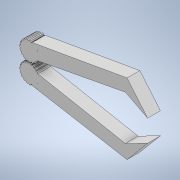
# Autodesk Inventor part: Claw(2 gear)
Saved by Autodesk Inventor 2021 (Build 250183000, 183)
## iProperties
Created: 2022-03-06
Part Number: Claw(2 gear)
Material: Generic
Document SubType Name: Modeling
Designer: Pradeep
Density: 1 g/cm^3
Appearance: Default
Author: Pradeep
Autodesk Inventor part; units mm, degrees
ref_plane "YZ Plane" through (0, 0, 0) normal (1, 0, 0) x (0, 1, 0)
ref_plane "XZ Plane" through (0, 0, 0) normal (0, 1, 0) x (-1, 0, 0)
ref_plane "XY Plane" through (0, 0, 0) normal (0, 0, 1) x (1, 0, 0)
sketch "Sketch1" plane through (0, 0, 0) normal (0, 0, 1) x (1, 0, 0)
  line L0 (36.6027, 32.7929) -> (34.9871, 31.7929)
  line L1 (34.9871, 29.7929) -> (34.9871, 31.7929)
  line L2 (34.9871, 29.7929) -> (36.6027, 28.7929)
  line L3 (36.6767, 28.3494) -> (35.4733, 26.879)
  line L4 (36.1227, 24.9874) -> (35.4733, 26.879)
  line L5 (36.1227, 24.9874) -> (37.9755, 24.5661)
  line L6 (38.1895, 24.1708) -> (37.5287, 22.3893)
  line L7 (38.7572, 20.811) -> (37.5287, 22.3893)
  line L8 (38.7572, 20.811) -> (40.6463, 21.0142)
  line L9 (40.9771, 20.7097) -> (40.9306, 18.8102)
  line L10 (42.6049, 17.7163) -> (40.9306, 18.8102)
  line L11 (42.6049, 17.7163) -> (44.3257, 18.5219)
  line L12 (44.7374, 18.3413) -> (45.3102, 16.5297)
  line L13 (47.249, 16.0387) -> (45.3102, 16.5297)
  line L14 (47.249, 16.0387) -> (48.615, 17.3594)
  line L15 (49.0631, 17.3223) -> (50.1931, 15.7948)
  line L16 (52.1862, 15.9599) -> (50.1931, 15.7948)
  line L17 (52.1862, 15.9599) -> (53.0494, 17.6526)
  line L18 (53.4852, 17.7629) -> (55.05, 16.6851)
  line L19 (56.8815, 17.4885) -> (55.05, 16.6851)
  line L20 (56.8815, 17.4885) -> (57.1483, 19.3697)
  line L21 (57.5247, 19.6156) -> (59.3546, 19.1043)
  line L22 (60.8261, 20.4588) -> (59.3546, 19.1043)
  line L23 (60.8261, 20.4588) -> (60.4676, 22.3247)
  line L24 (60.7437, 22.6795) -> (62.6405, 22.79)
  line L25 (63.5924, 24.549) -> (62.6405, 22.79)
  line L26 (63.5924, 24.549) -> (62.6475, 26.1974)
  line L27 (62.7935, 26.6226) -> (64.5516, 27.3431)
  line L28 (64.8808, 29.3158) -> (64.5516, 27.3431)
  line L29 (64.8808, 29.3158) -> (63.4519, 30.5681)
  line L30 (63.4519, 31.0176) -> (64.8808, 32.2699)
  line L31 (64.5516, 34.2426) -> (64.8808, 32.2699)
  line L32 (64.5516, 34.2426) -> (62.7935, 34.9631)
  line L33 (62.6475, 35.3883) -> (63.5924, 37.0367)
  line L34 (62.6405, 38.7957) -> (63.5924, 37.0367)
  line L35 (62.6405, 38.7957) -> (60.7437, 38.9062)
  line L36 (60.4676, 39.261) -> (60.8261, 41.1269)
  line L37 (59.3546, 42.4814) -> (60.8261, 41.1269)
  line L38 (59.3546, 42.4814) -> (57.5247, 41.9701)
  line L39 (57.1483, 42.216) -> (56.8815, 44.0972)
  line L40 (55.05, 44.9006) -> (56.8815, 44.0972)
  line L41 (55.05, 44.9006) -> (53.4852, 43.8228)
  line L42 (53.0494, 43.9331) -> (52.1862, 45.6258)
  line L43 (50.1931, 45.7909) -> (52.1862, 45.6258)
  line L44 (50.1931, 45.7909) -> (49.0631, 44.2634)
  line L45 (48.615, 44.2263) -> (47.249, 45.547)
  line L46 (45.3102, 45.056) -> (47.249, 45.547)
  line L47 (45.3102, 45.056) -> (44.7374, 43.2444)
  line L48 (44.3257, 43.0638) -> (42.6049, 43.8694)
  line L49 (40.9306, 42.7755) -> (42.6049, 43.8694)
  line L50 (40.9306, 42.7755) -> (40.9771, 40.876)
  line L51 (40.6463, 40.5715) -> (38.7572, 40.7747)
  line L52 (37.5287, 39.1964) -> (38.7572, 40.7747)
  line L53 (37.5287, 39.1964) -> (38.1895, 37.4149)
  line L54 (37.9755, 37.0196) -> (36.1227, 36.5983)
  line L55 (35.4733, 34.7067) -> (36.1227, 36.5983)
  line L56 (35.4733, 34.7067) -> (36.6767, 33.2363)
  arc A0 (40.9771, 40.876) -> (40.6463, 40.5715) centre (49.9537, 30.7929) ccw
  arc A1 (44.7374, 43.2444) -> (44.3257, 43.0638) centre (49.9537, 30.7929) ccw
  arc A2 (49.0631, 44.2634) -> (48.615, 44.2263) centre (49.9537, 30.7929) ccw
  arc A3 (53.4852, 43.8228) -> (53.0494, 43.9331) centre (49.9537, 30.7929) ccw
  arc A4 (57.5247, 41.9701) -> (57.1483, 42.216) centre (49.9537, 30.7929) ccw
  arc A5 (60.7437, 38.9062) -> (60.4676, 39.261) centre (49.9537, 30.7929) ccw
  arc A6 (62.7935, 34.9631) -> (62.6475, 35.3883) centre (49.9537, 30.7929) ccw
  arc A7 (63.4519, 30.5681) -> (63.4519, 31.0176) centre (49.9537, 30.7929) ccw
  arc A8 (62.6475, 26.1974) -> (62.7935, 26.6226) centre (49.9537, 30.7929) ccw
  arc A9 (60.4676, 22.3247) -> (60.7437, 22.6795) centre (49.9537, 30.7929) ccw
  arc A10 (57.1483, 19.3697) -> (57.5247, 19.6156) centre (49.9537, 30.7929) ccw
  arc A11 (53.0494, 17.6526) -> (53.4852, 17.7629) centre (49.9537, 30.7929) ccw
  arc A12 (48.615, 17.3594) -> (49.0631, 17.3223) centre (49.9537, 30.7929) ccw
  arc A13 (44.3257, 18.5219) -> (44.7374, 18.3413) centre (49.9537, 30.7929) ccw
  arc A14 (40.6463, 21.0142) -> (40.9771, 20.7097) centre (49.9537, 30.7929) ccw
  arc A15 (37.9755, 24.5661) -> (38.1895, 24.1708) centre (49.9537, 30.7929) ccw
  arc A16 (36.6027, 28.7929) -> (36.6767, 28.3494) centre (49.9537, 30.7929) ccw
  arc A17 (38.1895, 37.4149) -> (37.9755, 37.0196) centre (49.9537, 30.7929) ccw
  arc A18 (36.6767, 33.2363) -> (36.6027, 32.7929) centre (49.9537, 30.7929) ccw
  arc A19 (37.5287, 22.3893) -> (38.2823, 21.3706) centre (49.9537, 30.7929) ccw
  arc A20 (63.5924, 37.0367) -> (62.6405, 38.7957) centre (49.9537, 30.7929) ccw
  arc A21 (41.5275, 43.2025) -> (40.9306, 42.7755) centre (49.9537, 30.7929) ccw
  line L57 (55.05, 44.9006) -> (202.7711, 70.9478)
  line L58 (202.7711, 70.9478) -> (234.9105, 32.6456)
  line L59 (234.9105, 32.6456) -> (200.2006, 50.4283)
  line L60 (200.2006, 50.4283) -> (63.5924, 24.549)
  line L61 (36.6027, -1.389) -> (34.9871, -0.389)
  line L62 (34.9871, 1.611) -> (34.9871, -0.389)
  line L63 (34.9871, 1.611) -> (36.6027, 2.611)
  line L64 (36.6767, 3.0545) -> (35.4733, 4.5249)
  line L65 (36.1227, 6.4165) -> (35.4733, 4.5249)
  line L66 (36.1227, 6.4165) -> (37.9755, 6.8378)
  line L67 (38.1895, 7.2331) -> (37.5287, 9.0146)
  line L68 (38.7572, 10.5929) -> (37.5287, 9.0146)
  line L69 (38.7572, 10.5929) -> (40.6463, 10.3897)
  line L70 (40.9771, 10.6942) -> (40.9306, 12.5937)
  line L71 (42.6049, 13.6876) -> (40.9306, 12.5937)
  line L72 (42.6049, 13.6876) -> (44.3257, 12.882)
  line L73 (44.7374, 13.0626) -> (45.3102, 14.8742)
  line L74 (47.249, 15.3652) -> (45.3102, 14.8742)
  line L75 (47.249, 15.3652) -> (48.615, 14.0445)
  line L76 (49.0631, 14.0816) -> (50.1931, 15.6091)
  line L77 (52.1862, 15.444) -> (50.1931, 15.6091)
  line L78 (52.1862, 15.444) -> (53.0494, 13.7513)
  line L79 (53.4852, 13.641) -> (55.05, 14.7188)
  line L80 (56.8815, 13.9154) -> (55.05, 14.7188)
  line L81 (56.8815, 13.9154) -> (57.1483, 12.0342)
  line L82 (57.5247, 11.7883) -> (59.3546, 12.2996)
  line L83 (60.8261, 10.9451) -> (59.3546, 12.2996)
  line L84 (60.8261, 10.9451) -> (60.4676, 9.0792)
  line L85 (60.7437, 8.7244) -> (62.6405, 8.6138)
  line L86 (63.5924, 6.8549) -> (62.6405, 8.6138)
  line L87 (63.5924, 6.8549) -> (62.6475, 5.2065)
  line L88 (62.7935, 4.7813) -> (64.5516, 4.0608)
  line L89 (64.8808, 2.0881) -> (64.5516, 4.0608)
  line L90 (64.8808, 2.0881) -> (63.4519, 0.8358)
  line L91 (63.4519, 0.3863) -> (64.8808, -0.866)
  line L92 (64.5516, -2.8387) -> (64.8808, -0.866)
  line L93 (64.5516, -2.8387) -> (62.7935, -3.5592)
  line L94 (62.6475, -3.9844) -> (63.5924, -5.6328)
  line L95 (62.6405, -7.3918) -> (63.5924, -5.6328)
  line L96 (62.6405, -7.3918) -> (60.7437, -7.5023)
  line L97 (60.4676, -7.8571) -> (60.8261, -9.723)
  line L98 (59.3546, -11.0775) -> (60.8261, -9.723)
  line L99 (59.3546, -11.0775) -> (57.5247, -10.5662)
  line L100 (57.1483, -10.8121) -> (56.8815, -12.6933)
  line L101 (55.05, -13.4967) -> (56.8815, -12.6933)
  line L102 (55.05, -13.4967) -> (53.4852, -12.4189)
  line L103 (53.0494, -12.5292) -> (52.1862, -14.2219)
  line L104 (50.1931, -14.387) -> (52.1862, -14.2219)
  line L105 (50.1931, -14.387) -> (49.0631, -12.8595)
  line L106 (48.615, -12.8224) -> (47.249, -14.1431)
  line L107 (45.3102, -13.6521) -> (47.249, -14.1431)
  line L108 (45.3102, -13.6521) -> (44.7374, -11.8405)
  line L109 (44.3257, -11.6599) -> (42.6049, -12.4655)
  line L110 (40.9306, -11.3716) -> (42.6049, -12.4655)
  line L111 (40.9306, -11.3716) -> (40.9771, -9.4721)
  line L112 (40.6463, -9.1676) -> (38.7572, -9.3708)
  line L113 (37.5287, -7.7925) -> (38.7572, -9.3708)
  line L114 (37.5287, -7.7925) -> (38.1895, -6.011)
  line L115 (37.9755, -5.6157) -> (36.1227, -5.1944)
  line L116 (35.4733, -3.3028) -> (36.1227, -5.1944)
  line L117 (35.4733, -3.3028) -> (36.6767, -1.8324)
  arc A22 (40.6463, -9.1676) -> (40.9771, -9.4721) centre (49.9537, 0.611) ccw
  arc A23 (44.3257, -11.6599) -> (44.7374, -11.8405) centre (49.9537, 0.611) ccw
  arc A24 (48.615, -12.8224) -> (49.0631, -12.8595) centre (49.9537, 0.611) ccw
  arc A25 (53.0494, -12.5292) -> (53.4852, -12.4189) centre (49.9537, 0.611) ccw
  arc A26 (57.1483, -10.8121) -> (57.5247, -10.5662) centre (49.9537, 0.611) ccw
  arc A27 (60.4676, -7.8571) -> (60.7437, -7.5023) centre (49.9537, 0.611) ccw
  arc A28 (62.6475, -3.9844) -> (62.7935, -3.5592) centre (49.9537, 0.611) ccw
  arc A29 (63.4519, 0.3863) -> (63.4519, 0.8358) centre (49.9537, 0.611) ccw
  arc A30 (62.7935, 4.7813) -> (62.6475, 5.2065) centre (49.9537, 0.611) ccw
  arc A31 (60.7437, 8.7244) -> (60.4676, 9.0792) centre (49.9537, 0.611) ccw
  arc A32 (57.5247, 11.7883) -> (57.1483, 12.0342) centre (49.9537, 0.611) ccw
  arc A33 (53.4852, 13.641) -> (53.0494, 13.7513) centre (49.9537, 0.611) ccw
  arc A34 (49.0631, 14.0816) -> (48.615, 14.0445) centre (49.9537, 0.611) ccw
  arc A35 (44.7374, 13.0626) -> (44.3257, 12.882) centre (49.9537, 0.611) ccw
  arc A36 (40.9771, 10.6942) -> (40.6463, 10.3897) centre (49.9537, 0.611) ccw
  arc A37 (38.1895, 7.2331) -> (37.9755, 6.8378) centre (49.9537, 0.611) ccw
  arc A38 (36.6767, 3.0545) -> (36.6027, 2.611) centre (49.9537, 0.611) ccw
  arc A39 (37.9755, -5.6157) -> (38.1895, -6.011) centre (49.9537, 0.611) ccw
  arc A40 (36.6027, -1.389) -> (36.6767, -1.8324) centre (49.9537, 0.611) ccw
  arc A41 (38.2823, 10.0333) -> (37.5287, 9.0146) centre (49.9537, 0.611) ccw
  arc A42 (62.6405, -7.3918) -> (63.5924, -5.6328) centre (49.9537, 0.611) ccw
  arc A43 (40.9306, -11.3716) -> (41.5275, -11.7986) centre (49.9537, 0.611) ccw
  line L118 (55.05, -13.4967) -> (202.7711, -39.5439)
  line L119 (202.7711, -39.5439) -> (234.9105, -1.2417)
  line L120 (234.9105, -1.2417) -> (200.2006, -19.0244)
  line L121 (200.2006, -19.0244) -> (63.5924, 6.8549)
  arc A44 (51.277, 15.8513) -> (51.458, 15.8685) centre (49.9537, 30.7929) ccw
  arc A45 (50.1931, 15.7948) -> (50.3325, 15.7976) centre (49.9537, 30.7929) ccw
  arc A46 (50.9264, 15.8244) -> (51.1394, 15.8398) centre (49.9537, 30.7929) ccw
  point P0 (0, 0)
  point P1 (60.3076, 11.4645)
  dimension "d8" = 360
  constraints: 244 end point, 94 point on circle, 47 centre point, 10 point on line, 2 coincident, 134 other
extrude "Extrusion1" add sketch "Sketch1" along normal blind 20 contours A18 L56 L55 L54 A17 L53 L52 L51 A0 L50 L49 L48 A1 L47 L46 L45 A2 L44 L43 L42 A3 L41 L40 L39 A4 L38 L37 L36 A5 L35 L34 L33 A6 L32 L31 L30 A7 L29 L28 L27 A8 L26 L25 L24 A9 L23 L22 L21 A10 L20 L19 L18 A11 L17 L16 L15 A12 L14 L13 L12 A13 L11 L10 L9 A14 L8 L7 L6 A15 L5 L4 L3 A16 L2 L1 L0 | L57 L58 L59 L60 L26 A8 L27 L28 L29 A7 L30 L31 L32 A6 L33 A20 L35 A5 L36 L37 L38 A4 L39 L40 | L61 L62 L63 A38 L64 L65 L66 A37 L67 L68 L69 A36 L70 L71 L72 A35 L73 L74 L75 A34 L76 L77 L78 A33 L79 L80 L81 A32 L82 L83 L84 A31 L85 L86 L87 A30 L88 L89 L90 A29 L91 L92 L93 A28 L94 L95 L96 A27 L97 L98 L99 A26 L100 L101 L102 A25 L103 L104 L105 A24 L106 L107 L108 A23 L109 L110 L111 A22 L112 L113 L114 A39 L115 L116 L117 A40 | L101 L100 A26 L99 L98 L97 A27 L96 A42 L94 A28 L93 L92 L91 A29 L90 L89 L88 A30 L87 L121 L120 L119 L118
body "Solid1"
